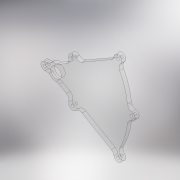
# Autodesk Inventor part: RailBaseBottom
Saved by Autodesk Inventor 2018.2 (Build 222227000, 227)
## iProperties
Created: 2018-03-27
Part Number: RailBaseBottom
Material: Polycarbonate, Clear
Document SubType Name: Modeling
Designer: mansu
Density: 1.2 g/cm^3
Appearance: Polycarbonate - Clear
Author: mansu
Autodesk Inventor part; units mm, degrees
ref_plane "YZ Plane" through (0, 0, 0) normal (1, 0, 0) x (0, 1, 0)
ref_plane "XZ Plane" through (0, 0, 0) normal (0, 1, 0) x (-1, 0, 0)
ref_plane "XY Plane" through (0, 0, 0) normal (0, 0, 1) x (1, 0, 0)
sketch "Sketch1" plane through (0, 0, 0) normal (0, 1, 0) x (-1, 0, 0)
  circle A0 centre (0, 0) radius 8
  arc A1 (-82.4777, 58.296) -> (-82.4777, -58.296) centre (0, 0) ccw construction
  arc A2 (-86.8253, 60.806) -> (-86.8253, -60.806) centre (0, 0) ccw construction
  arc A3 (-2, -11.8322) -> (-2, 11.8322) centre (0, 0) ccw
  line L0 (-2, -11.8322) -> (-89.433, -62.3116)
  arc A4 (-89.433, 62.3116) -> (-89.433, -62.3116) centre (0, 0) ccw
  line L1 (-2, 11.8322) -> (-89.433, 62.3116)
  circle A5 centre (-93.7631, -64.8116) radius 2
  circle A6 centre (-93.7631, 64.8116) radius 2
  circle A7 centre (-114, 0) radius 2
  circle A8 centre (-25, -30.8847) radius 2
  circle A9 centre (-25, 30.8847) radius 2
  circle A10 centre (17, 0) radius 2
  line L2 (10.3923, -6) -> (17, -6)
  arc A11 (17, -6) -> (17, 6) centre (17, 0) ccw
  line L3 (17, 6) -> (10.3923, 6)
  line L4 (-22.3038, -23.5546) -> (-19.8038, -27.8847)
  arc A12 (-30.1962, -33.8847) -> (-19.8038, -27.8847) centre (-25, -30.8847) ccw
  line L5 (-30.1962, -33.8847) -> (-32.6962, -29.5546)
  line L6 (-22.3038, 23.5546) -> (-19.8038, 27.8847)
  arc A13 (-19.8038, 27.8847) -> (-30.1962, 33.8847) centre (-25, 30.8847) ccw
  line L7 (-30.1962, 33.8847) -> (-32.6962, 29.5546)
  line L8 (-92.8025, 57.1726) -> (-96.9102, 59.7032)
  arc A14 (-88.567, 61.8116) -> (-96.9102, 59.7032) centre (-93.7631, 64.8116) ccw
  line L9 (-108.8347, -6) -> (-114, -6)
  arc A15 (-114, 6) -> (-114, -6) centre (-114, 0) ccw
  line L10 (-114, 6) -> (-108.8347, 6)
  line L11 (-92.8025, -57.1726) -> (-96.9102, -59.7032)
  arc A16 (-96.9102, -59.7032) -> (-88.567, -61.8116) centre (-93.7631, -64.8116) ccw
  point P0 (-109, 0)
  point P1 (12, 0)
  dimension "d0" = 16
  dimension "d1" = 101
  dimension "d3" = 12
  dimension "d6" = 60
  dimension "d7" = 2
  dimension "d8" = 5
  dimension "d9" = 3
  dimension "d10" = 4
  dimension "d12" = 5
  dimension "d13" = 5
  dimension "d14" = 5
  dimension "d15" = 5
  dimension "d16" = 5
  dimension "d17" = 5
  dimension "d18" = 25
  dimension "d19" = 6
  dimension "d20" = 6
  constraints: 28 point on circle, 24 end point, 17 centre point, 12 point on line, 10 concentric, 10 tangent, 9 equal radius, 3 horizontal alignment, 3 parallel, 3 perpendicular, 2 horizontal, 2 line through centre, 2 vertical alignment, 1 coincident
  measures "d0" diameter of A0
  measures "d1" radius of A1
  measures "d3" radius of A3
  measures "d6" angle of L1 L0
  measures "d7" horizontal distance of point (0, 0) L0.start
  measures "d8" radial gap between concentric circles of A1 A2
  measures "d9" radial gap between concentric circles of A2 A4
  measures "d10" diameter of A7
  measures "d12" distance of point (-109, 0) A7.centre
  measures "d13" distance of A10.centre point (12, 0)
  measures "d14" distance of L1.end A6.centre
  measures "d15" distance of A5.centre L0.end
  measures "d16" distance from line of L1 A9.centre
  measures "d17" distance from line of L0 A8.centre
  measures "d18" horizontal distance of A9.centre point (0, 0)
  measures "d19" radius of A11
  measures "d20" radius of A16
extrude "Extrusion1" add sketch "Sketch1" along normal blind 6 contours L0 A4 L1 A3
extrude "Extrusion2" add sketch "Sketch1" along normal blind 6 contours A3 L3 A11 L2 | L4 A12 L5 L0 | A16 L11 A4 L0 | L1 L7 A13 L6 | L1 A4 L8 A14 | L9 A15 L10 A4
fillet "Fillet1" radius 8 12 edges at (32.6962, 3, 29.5546) (22.3038, 3, 23.5546) (88.567, 3, 61.8116) (92.8025, 3, 57.1726) (108.8347, 3, -6) (108.8347, 3, 6) (92.8025, 3, -57.1726) (88.567, 3, -61.8116) (32.6962, 3, -29.5546) (22.3038, 3, -23.5546) (2, 3, -11.8322) (-10.3923, 3, 6)
body "Solid1"
